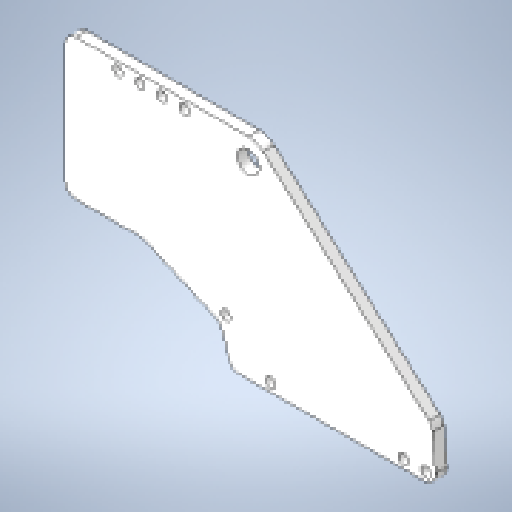
# Autodesk Inventor part: Uprights
Saved by Autodesk Inventor 2023.2 (Build 272271000, 271)
## iProperties
Created: 2024-02-11
Part Number: Uprights
Material: UHMW, White
Document SubType Name: Modeling
Designer: Nathan Cai
Density: 0.94 g/cm^3
Appearance: Smooth - White
Mass: 5.62646 g
Surface Area: 31.1778 cm^2
Volume: 5.98559 cm^3
Author: Nathan Cai
Autodesk Inventor part; units mm, degrees
ref_plane "YZ Plane" through (0, 0, 0) normal (1, 0, 0) x (0, 1, 0)
ref_plane "XZ Plane" through (0, 0, 0) normal (0, 1, 0) x (-1, 0, 0)
ref_plane "XY Plane" through (0, 0, 0) normal (0, 0, 1) x (1, 0, 0)
sketch "Sketch1" plane through (0, 0, 0) normal (0, 0, 1) x (1, 0, 0)
  line L0 (0, 0) -> (0, 136.525)
  line L1 (-11.7886, 12.2907) -> (-39.6863, 18.4755) construction
  line L2 (-39.6863, 18.4755) -> (-33.3297, 47.1481) construction
  line L3 (-33.3297, 47.1481) -> (-5.432, 40.9633) construction
  line L4 (-5.432, 40.9633) -> (-11.7886, 12.2907) construction
  line L5 (-39.6863, 18.4755) -> (-5.432, 40.9633) construction
  line L6 (-33.3297, 47.1481) -> (-11.7886, 12.2907) construction
  circle A0 centre (-53.975, 12.7) radius 3.175
  circle A1 centre (-53.975, 12.7) radius 6.35
  line L7 (0, 0) -> (-54.712, 6.3929) construction
  line L8 (-59.6703, 15.5082) -> (0, 136.525) construction
  line L9 (-27.1302, 45.7737) -> (-37.4529, 28.5497) construction
  line L10 (-11.6315, 42.3377) -> (-9.5552, 22.3649) construction
  line L11 (-19.3809, 44.0557) -> (-25.7374, 15.3831) construction
  line L12 (0, 92.075) -> (-19.7574, 96.4551) construction
  line L13 (-35.3766, 8.5768) -> (-19.8779, 5.1408) construction
  line L14 (-19.8779, 5.1408) -> (-21.2523, -1.0586) construction
  line L15 (-21.2523, -1.0586) -> (-36.751, 2.3773) construction
  line L16 (-36.751, 2.3773) -> (-35.3766, 8.5768) construction
  line L17 (-35.3766, 8.5768) -> (-41.27, 4.8223) construction
  line L18 (-19.8779, 5.1408) -> (-17.9381, 2.096) construction
  line L19 (-5.432, 40.9633) -> (-33.3297, 47.1481) construction
  line L20 (-33.3297, 47.1481) -> (-32.2475, 52.0296) construction
  line L21 (-32.2475, 52.0296) -> (-4.3498, 45.8448) construction
  line L22 (-4.3498, 45.8448) -> (-5.432, 40.9633) construction
  line L23 (-53.2878, 15.7997) -> (-53.975, 12.7) construction
  line L24 (-53.975, 12.7) -> (-57.0747, 13.3872) construction
  line L25 (-27.6272, 6.8588) -> (-34.4992, -24.1386) construction
  line L26 (-31.8676, 50.076) -> (-5.5198, 44.2349) construction
  line L27 (-5.5198, 44.2349) -> (-4.489, 48.8845) construction
  line L28 (-4.489, 48.8845) -> (-30.8368, 54.7256) construction
  line L29 (-30.8368, 54.7256) -> (-31.8676, 50.076) construction
  line L30 (-31.3522, 52.4008) -> (-5.0044, 46.5597) construction
  circle A2 centre (-29.0274, 51.8854) radius 1.4732 construction
  circle A3 centre (-22.8279, 50.5111) radius 1.4732 construction
  circle A4 centre (-16.6284, 49.1367) radius 1.4732 construction
  circle A5 centre (-10.4289, 47.7623) radius 1.4732 construction
  circle A6 centre (-10.3614, 84.7398) radius 1.4732 construction
  line L31 (-53.975, 12.7) -> (-13.3751, 95.0402) construction
  line L32 (-32.2923, 56.6744) -> (0, 49.5153) construction
  circle A7 centre (-10.3614, 84.7398) radius 4.7625 construction
  line L33 (-4.7625, 50.5712) -> (-4.7625, 93.1308) construction
  line L34 (-27.5056, 55.6132) -> (-14.3936, 82.2055) construction
  line L35 (-5.6003, 84.6261) -> (-4.7625, 84.4403) construction
  line L36 (-17.9381, 2.096) -> (0, 2.096) construction
  line L37 (0, 2.096) -> (0, -1.079) construction
  line L38 (0, -1.079) -> (-17.9381, -1.079) construction
  line L39 (-17.9381, -1.079) -> (-17.9381, 2.096) construction
  circle A8 centre (-12.7, 7.9375) radius 1.5875 construction
  line L40 (-12.7, 7.9375) -> (0, 7.9375) construction
  line L41 (0, 7.9375) -> (-17.9381, 2.096)
  circle A9 centre (-12.7, 7.9375) radius 3.175 construction
  line L42 (-9.525, 7.9375) -> (-9.525, 4.8357) construction
  line L43 (-9.525, 7.9375) -> (0, 7.9375) construction
  line L44 (-17.9187, 46.9837) -> (-16.8879, 51.6333) construction
  line L45 (-12.4942, 45.7811) -> (-26.2381, -16.2137) construction
  line L46 (0, 66.675) -> (0, 7.9375) construction
  line L47 (-26.2381, -16.2137) -> (-20.0386, -17.5881) construction
  line L48 (-20.0386, -17.5881) -> (-8.7313, 7.9375)
  circle A10 centre (-12.7, 6.35) radius 1.4224
  line L49 (0, 13.4938) -> (-4.7625, 13.4938) construction
  line L50 (-4.7625, 13.4938) -> (-4.7625, 24.6063) construction
  line L51 (-4.7625, 24.6063) -> (0, 24.6063) construction
  line L52 (0, 24.6063) -> (0, 13.4938) construction
  line L53 (-4.7625, 19.05) -> (0, 19.05) construction
  circle A11 centre (-2.3813, 19.05) radius 1.4224
  line L54 (-20.7405, 8.5842) -> (-9.7454, 58.18) construction
  line L55 (-9.7454, 58.18) -> (-3.5459, 56.8056) construction
  line L56 (-3.5459, 56.8056) -> (-14.5411, 7.2098) construction
  line L57 (-14.5411, 7.2098) -> (-20.7405, 8.5842) construction
  line L58 (-12.7, 6.35) -> (-12.7, 7.9375) construction
  line L59 (-11.5442, 1.5875) -> (-9.525, 1.5875) construction
  line L60 (-9.525, 1.5875) -> (-9.525, 7.9375) construction
  line L61 (-9.525, 7.9375) -> (-11.5442, 7.9375) construction
  line L62 (-11.5442, 7.9375) -> (-11.5442, 1.5875) construction
  line L63 (-9.7454, 58.18) -> (-15.9449, 59.5544) construction
  line L64 (-15.9449, 59.5544) -> (-14.6504, 65.3933) construction
  line L65 (-14.6504, 65.3933) -> (0, 66.675)
  line L66 (-9.7454, 58.18) -> (-17.3193, 53.3549) construction
  arc A12 (-10.2313, 55.9882) -> (-11.9373, 58.6659) centre (-11.0843, 57.3271) ccw construction
  line L67 (-4.7625, 57.15) -> (0, 57.15) construction
  circle A13 centre (-2.3813, 57.15) radius 1.4224
  circle A14 centre (-2.3813, 63.5) radius 1.4224
  line L68 (0, 7.9375) -> (-60.325, 7.9375) construction
  line L69 (-60.325, 7.9375) -> (-60.325, -39.6875) construction
  line L70 (-60.325, -39.6875) -> (0, -39.6875)
  line L71 (0, -39.6875) -> (0, 7.9375)
  line L72 (-60.325, -39.6875) -> (-60.325, 12.7)
  line L73 (-58.6735, 16.9717) -> (-14.6504, 65.3933)
  line L74 (-60.325, -30.1625) -> (-60.325, -3.175) construction
  line L75 (-60.325, -3.175) -> (-55.5625, -3.175) construction
  line L76 (-55.5625, -3.175) -> (-55.5625, -30.1625) construction
  line L77 (-55.5625, -30.1625) -> (-60.325, -30.1625) construction
  line L78 (-60.325, -24.6062) -> (-55.5625, -24.6062) construction
  circle A15 centre (-57.9437, -24.6063) radius 1.4224
  circle A16 centre (-57.9437, -18.2563) radius 1.4224
  circle A17 centre (-57.9437, -11.9063) radius 1.4224
  circle A18 centre (-57.9437, -5.5563) radius 1.4224
  line L79 (-20.0386, -17.5881) -> (-20.0386, -39.6875)
  point P0 (-22.5591, 29.7194)
  point P1 (-20.4869, 2.3938)
  point P2 (-36.3367, 4.2458)
  point P3 (-51.1668, 18.3953)
  point P4 (-11.1125, 7.9375)
  point P5 (-11.4283, 6.9872)
  point P6 (-11.9574, 7.9375)
  point P7 (-13.9717, 6.9872)
  point P8 (-9.525, 6.1457)
  point P9 (-10.2031, 4.6149)
  dimension "d74" = 6.35
  dimension "d13" = 136.525
  dimension "d14" = 29.3687
  dimension "d15" = 28.575
  dimension "d16" = 12.5
  dimension "d17" = 6.35
  dimension "d19" = 53.975
  dimension "d22" = 12.7
  dimension "d23" = 7.9375
  dimension "d24" = 19.05
  dimension "d26" = 102.5
  dimension "d29" = 6.35
  dimension "d31" = 7.9375
  dimension "d34" = 5
  dimension "d35" = 26.9875
  dimension "d38" = 31.75
  dimension "d40" = 26.9875
  dimension "d41" = 4.7625
  dimension "d42" = 2.9464
  dimension "d43" = 2.3813
  dimension "d46" = 6.35
  dimension "d51" = 2.9464
  dimension "d52" = 79.7719
  dimension "d53" = 6.35
  dimension "d54" = 9.525
  dimension "d55" = 4.7625
  dimension "d56" = 4.7625
  dimension "d60" = 12.7
  dimension "d61" = 3.175
  dimension "d63" = 3.175
  dimension "d66" = 3.175
  dimension "d67" = 12.7
  dimension "d72" = 8.7312
  dimension "d73" = 7.9375
  dimension "d75" = 34.925
  dimension "d80" = 12.7
  dimension "d82" = 7.9375
  dimension "d83" = 63.5
  dimension "d84" = 66.675
  dimension "d85" = 6.35
  dimension "d86" = 92.075
  dimension "d87" = 2.8448
  dimension "d88" = 4.7625
  dimension "d89" = 11.1125
  dimension "d90" = 2.8448
  dimension "d91" = 19.05
  dimension "d92" = 6.35
  dimension "d93" = 50.8
  dimension "d94" = 25.4
  dimension "d95" = 8.7312
  dimension "d96" = 9.525
  dimension "d97" = 6.35
  dimension "d99" = 6.35
  dimension "d101" = 3.175
  dimension "d106" = 2.8448
  dimension "d107" = 57.15
  dimension "d110" = 6.35
  dimension "d119" = 85
  dimension "d121" = 47.625
  dimension "d123" = 4.7625
  dimension "d124" = 26.9875
  dimension "d125" = 9.525
  dimension "d126" = 2.8448
  dimension "d130" = 6.35
  dimension "d135" = 2.3813
  constraints: 160 end point, 46 point on line, 29 parallel, 22 perpendicular, 18 centre point, 13 point on circle, 11 midpoint, 10 coincident, 6 vertical, 4 horizontal, 4 tangent, 2 collinear, 1 horizontal alignment, 22 other
  measures "d13" distance of L0.start L0.end
  measures "d14" distance of L1.end L2.end
  measures "d15" distance between parallel lines of L4 L2
  measures "d16" angle of L0 L4
  measures "d17" diameter of A0
  measures "d19" distance from line of L0 A0.centre
  measures "d22" diameter of A1
  measures "d23" distance from line of L9.start L11
  measures "d24" distance from line of L9.end L3
  measures "d26" angle of L0 L12
  measures "d29" distance of L13.end L14.end
  measures "d31" distance between parallel lines of L14 L11
  measures "d34" distance of L2.end L20.end
  measures "d35" distance between parallel lines of L11 L23
  measures "d38" distance of L25.start L25.end
  measures "d40" distance between parallel lines of L27 L29
  measures "d41" distance between parallel lines of L26 L28
  measures "d42" diameter of A2
  measures "d43" distance from line of L29 A2.centre
  measures "d46" distance of A2.centre A3.centre
  measures "d51" diameter of A6
  measures "d52" distance from line of L13 A6.centre
  measures "d53" distance between parallel lines of L32 L26
  measures "d54" diameter of A7
  measures "d55" distance between parallel lines of L0 L33
  measures "d56" distance between parallel lines of L31 L34
  measures "d60" vertical distance of A0.centre L0.start
  measures "d61" distance between parallel lines of L3 L26
  measures "d63" distance between parallel lines of L36 L38
  measures "d66" diameter of A8
  measures "d67" distance from line of L0 A8.centre
  measures "d72" distance between parallel lines of L1 L13
  measures "d73" distance from line of L0.start L40
  measures "d75" vertical distance of point (0, 49.515) point (-4.763, 84.44)
  measures "d80" distance between parallel lines of L27 L44
  measures "d82" distance between parallel lines of L4 L45
  measures "d83" distance from line of L45.end L26
  measures "d84" distance of L0.start L46.start
  measures "d85" distance of L45.end L47.end
  measures "d86" distance of L0.start point (0, 92.075)
  measures "d87" diameter of A10
  measures "d88" distance of L50.end L51.end
  measures "d89" distance of L49.end L50.end
  measures "d90" diameter of A11
  measures "d91" distance from line of L0.start L53
  measures "d92" distance between parallel lines of L54 L56
  measures "d93" distance between parallel lines of L55 L57
  measures "d94" distance between parallel lines of L47 L57
  measures "d95" distance from line of L0 L48.end
  measures "d96" distance between parallel lines of L0 L60
  measures "d97" distance between parallel lines of L40 L59
  measures "d99" distance of L63.start L63.end
  measures "d101" diameter of A12
  measures "d106" diameter of A13
  measures "d107" distance from line of L0.start L67
  measures "d110" distance of A13.centre A14.centre
  measures "d119" angle of L0 L65
  measures "d121" distance of L69.end L68.end
  measures "d123" distance of L74.end L75.end
  measures "d124" distance between parallel lines of L77 L75
  measures "d125" distance from line of L69.end L77
  measures "d126" diameter of A15
  measures "d130" distance of A15.centre A16.centre
  measures "d135" distance from line of L75 A18.centre
extrude "Extrusion1" add sketch "Sketch1" along normal blind 3.175 contours L41 L48 L79 L70 L72 A1 L73 L65 L0 | A1
fillet "Fillet5" radius 3.175 6 edges at (-14.6504, 65.3933, 1.5875) (0, 66.675, 1.5875) (-20.0386, -39.6875, 1.5875) (-20.0386, -17.5881, 1.5875) (-10.2031, 4.6149, 1.5875) (0, 7.9375, 1.5875)
equation "\"d56\" = d55"
body "Solid1"
